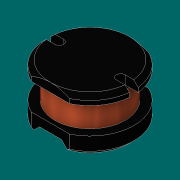
# Autodesk Inventor part: SDR0503
Saved by Autodesk Inventor 2016 (Build 200138000, 138)
## iProperties
Created: 2015-11-05
Part Number: SDR0503
Material: ABS Plastic
Document SubType Name: Modeling
Designer: Sawaiz
Density: 1.06 g/cm^3
Appearance: Smooth - Black
Author: Sawaiz
Autodesk Inventor part; units mm, degrees
ref_plane "YZ Plane" through (0, 0, 0) normal (1, 0, 0) x (0, 1, 0)
ref_plane "XZ Plane" through (0, 0, 0) normal (0, 1, 0) x (-1, 0, 0)
ref_plane "XY Plane" through (0, 0, 0) normal (0, 0, 1) x (1, 0, 0)
sketch "Sketch1" plane through (0, 0, 0) normal (0, 0, 1) x (1, 0, 0)
  circle A0 centre (0, 0) radius 2
  dimension "d0" = 4
  constraints: 1 centre point, 1 coincident
  measures "d0" diameter of A0
extrude "Extrusion1" add sketch "Sketch1" along normal blind 1.5
sketch "Sketch2" plane through (0, 0, 0) normal (0, 0, -1) x (-1, 0, 0)
  circle A0 centre (0, 0) radius 2.5
  dimension "d3" = 5
  constraints: 1 centre point, 1 coincident
  measures "d3" diameter of A0
extrude "Extrusion2" add sketch "Sketch2" along normal blind 1
sketch "Sketch3" plane through (0, 0, 1.5) normal (0, 0, 1) x (1, 0, 0)
  circle A0 centre (0, 0) radius 2.5
  dimension "d6" = 5
  constraints: 1 centre point, 1 coincident
  measures "d6" diameter of A0
extrude "Extrusion3" add sketch "Sketch3" along normal blind 0.5
chamfer "Chamfer1" distance 0.25 angle 45 2 edges at (-2.5, 0, 2) (2.5, 0, -1)
sketch "Sketch4" plane through (0, 0, 0) normal (1, 0, 0) x (0, 1, 0)
  line L0 (2.5, 0) -> (-2.5, 0) projected
  line L1 (-2.5, -1) -> (2.5, -1) projected
  line L2 (0, -1) -> (0, 0)
  line L3 (-1.125, -1) -> (-0.625, -0.5)
  line L4 (-0.625, -0.5) -> (0.625, -0.5)
  line L5 (0.625, -0.5) -> (1.125, -1)
  point P0 (0, -0.5)
  dimension "d14" = 1.25
  constraints: 8 end point, 3 midpoint, 2 point on line, 1 horizontal, 1 vertical
  measures "d14" distance of L3.end L4.end
extrude "Extrusion4" cut sketch "Sketch4" along normal through all both and the other way through all
sketch "Sketch5" plane through (0, 0, 2) normal (0, 0, 1) x (1, 0, 0)
  line L0 (-2.25, 5) -> (2.25, 5)
  line L1 (2.25, 5) -> (2.25, -5)
  line L2 (2.25, -5) -> (-2.25, -5)
  line L3 (-2.25, -5) -> (-2.25, 5)
  line L4 (-2.25, 5) -> (2.25, -5) construction
  line L5 (2.25, 5) -> (-2.25, -5) construction
  point P0 (0, 0)
  dimension "d18" = 4.5
  dimension "d19" = 10
  constraints: 12 end point, 2 midpoint, 2 parallel, 1 horizontal, 1 perpendicular
  measures "d18" distance of L1.end L2.end
  measures "d19" distance of L0.end L1.end
extrude "Extrusion5" cut sketch "Sketch5" along normal through all both and the other way through all keep common part
sketch "Sketch6" plane through (0, 0, 2) normal (0, 0, 1) x (1, 0, 0)
  arc A0 (-2.25, 0) -> (2.25, 0) centre (0, 0) ccw projected
  arc A1 (2.25, 0) -> (-2.25, 0) centre (0, 0) ccw projected
  arc A2 (1.9486, 1.125) -> (-1.9486, 1.125) centre (0, 0) ccw projected
  line L0 (0, 2.25) -> (0, -2.25)
  circle A3 centre (0, 1.75) radius 0.25
  arc A4 (2.25, 1.0897) -> (-2.25, 1.0897) centre (0, 0) ccw projected
  line L1 (0.25, 1.75) -> (0.25, 2.4875)
  arc A5 (2.25, 1.0897) -> (-2.25, 1.0897) centre (0, 0) ccw projected
  line L2 (-0.25, 1.75) -> (-0.25, 2.4875)
  dimension "d22" = 0.5
  dimension "d24" = 0.5
  constraints: 9 point on circle, 6 end point, 2 tangent, 2 vertical, 1 centre point, 1 point on line
  measures "d24" diameter of A3
extrude "Extrusion6" cut sketch "Sketch6" against normal up to surface (0.5 mm away) contours A3 L0 | L0 A3 | L2 A4 L1 A1 | A1 L0 A3 L2 | L0 A1 L1 A3
mirror "Mirror1" about plane through (0, 0, 0) normal (0, 1, 0) of "Extrusion6"
body "Solid1"
